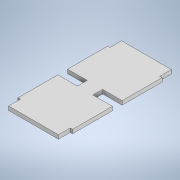
# Autodesk Inventor part: plate
Saved by Autodesk Inventor 2022 (Build 260153000, 153)
## iProperties
Created: 2023-04-13
Part Number: plate
Material: 一般
Document SubType Name: Modeling
Designer: Johnny Jou
Density: 1 g/cm^3
Appearance: 預設
Author: Johnny Jou
Autodesk Inventor part; units mm, degrees
ref_plane "YZ Plane" through (0, 0, 0) normal (1, 0, 0) x (0, 1, 0)
ref_plane "XZ Plane" through (0, 0, 0) normal (0, 1, 0) x (-1, 0, 0)
ref_plane "XY Plane" through (0, 0, 0) normal (0, 0, 1) x (1, 0, 0)
sketch "草圖1" plane through (0, 0, 0) normal (0, 1, 0) x (-1, 0, 0)
  line L0 (140, 0) -> (0, 0)
  line L1 (0, 0) -> (0, -290)
  line L2 (0, -290) -> (140, -290)
  line L3 (140, -290) -> (140, 0)
  line L4 (0, 0) -> (6, 0)
  line L5 (6, 0) -> (6, -30)
  line L6 (6, -30) -> (0, -30)
  line L7 (0, -30) -> (0, 0)
  line L8 (140, 0) -> (134, 0)
  line L9 (134, 0) -> (134, -30)
  line L10 (134, -30) -> (140, -30)
  line L11 (140, -30) -> (140, 0)
  line L12 (140, -290) -> (134, -290)
  line L13 (134, -290) -> (134, -260)
  line L14 (134, -260) -> (140, -260)
  line L15 (140, -260) -> (140, -290)
  line L16 (0, -290) -> (6, -290)
  line L17 (6, -290) -> (6, -260)
  line L18 (6, -260) -> (0, -260)
  line L19 (0, -260) -> (0, -290)
  line L20 (140, -132.5) -> (90, -132.5)
  line L21 (90, -132.5) -> (90, -157.5)
  line L22 (90, -157.5) -> (140, -157.5)
  line L23 (140, -157.5) -> (140, -132.5)
  line L24 (50, -132.5) -> (0, -132.5)
  line L25 (0, -132.5) -> (0, -157.5)
  line L26 (0, -157.5) -> (50, -157.5)
  line L27 (50, -157.5) -> (50, -132.5)
  point P0 (140, -145)
  point P1 (0, -145)
  dimension "d0" = 140
  dimension "d1" = 290
  dimension "d2" = 6
  dimension "d3" = 30
  dimension "d4" = 50
  dimension "d5" = 25
  constraints: 56 end point, 14 parallel, 7 equal length, 7 horizontal, 7 perpendicular, 4 midpoint, 1 coincident, 1 point on line
  measures "d0" distance between parallel lines of L1 L3
  measures "d1" distance between parallel lines of L2 L0
  measures "d2" distance of L5.end L6.end
  measures "d3" distance of L4.end L5.end
  measures "d4" distance of L20.start L20.end
  measures "d5" distance of L20.end L21.end
extrude "擠出1" add sketch "草圖1" along normal blind 10 contours L9 L10 L3 L20 L21 L22 L14 L13 L2 L17 L18 L1 L26 L27 L24 L6 L5 L0
